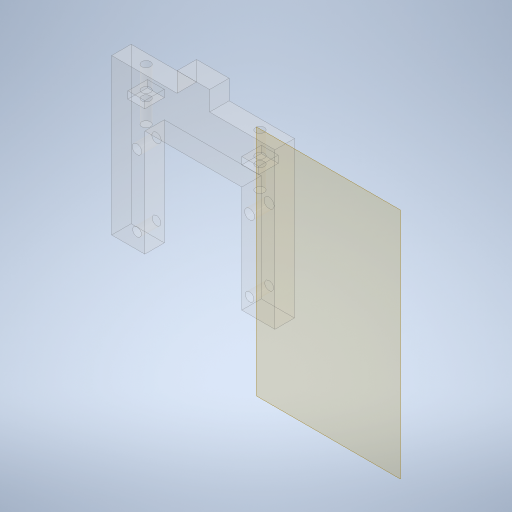
# Autodesk Inventor part: frame_knee_to_bridge
Saved by Autodesk Inventor 2024 (Build 280153000, 153)
## iProperties
Created: 2024-09-03
Part Number: frame_knee_to_bridge
Material: PMMA 플라스틱
Document SubType Name: Modeling
Designer: jmha0
Density: 1.188 g/cm^3
Appearance: 폴리카보네이트 - 선명
Mass: 4.02545 g
Surface Area: 28.6989 cm^2
Volume: 3.38842 cm^3
Author: jmha0
Autodesk Inventor part; units mm, degrees
ref_plane "YZ Plane" through (0, 0, 0) normal (1, 0, 0) x (0, 1, 0)
ref_plane "XZ Plane" through (0, 0, 0) normal (0, 1, 0) x (-1, 0, 0)
ref_plane "XY Plane" through (0, 0, 0) normal (0, 0, 1) x (1, 0, 0)
ref_plane "작업 평면1" through (0, 0, 0) normal (0, 0, 1) x (1, 0, 0)
sketch "스케치1" plane through (0, 0, 0) normal (0, 0, 1) x (1, 0, 0)
  line L0 (-20.1, 0.025) -> (-14.5, 0.025) projected
  line L1 (-20.1, -44.6) -> (-20.1, 8.5) projected
  line L2 (20.1, 0.025) -> (14.5, 0.025) projected
  line L3 (20.1, 8.5) -> (20.1, -44.6) projected
  circle A0 centre (17.3, 4) radius 1.45 projected
  circle A1 centre (-17.3, 4) radius 1.35 projected
  circle A2 centre (-17.3, 4) radius 1.45
  circle A3 centre (17.3, 4) radius 1.55
  line L4 (14.9, 0.025) -> (14.9, 15.025)
  line L5 (-14.9, 15.025) -> (-14.9, 0.025)
  line L6 (-20.1, 0.025) -> (-20.1, 15.025)
  line L7 (20.1, 0.025) -> (20.1, 15.025)
  line L8 (-20.1, 15.025) -> (20.1, 15.025)
  line L9 (-20.1, 0.025) -> (-14.9, 0.025)
  line L10 (14.9, 0.025) -> (20.1, 0.025)
  line L11 (-14.9, 0.025) -> (-14.9, 10.025)
  line L12 (-14.9, 10.025) -> (14.9, 10.025)
  line L13 (14.9, 0.025) -> (20.1, 0.025)
  point P0 (0, 0)
  point P1 (-20.1, 8.5)
  point P2 (-14.9, 0.025)
  dimension "d0" = 0.1
  dimension "d1" = 0.1
  dimension "d4" = 15
  dimension "d5" = 15
  dimension "d9" = 10
  constraints: 20 end point, 5 point on line, 2 centre point, 2 collinear, 2 perpendicular, 1 vertical
  measures "d0" radial gap between concentric circles of A1 A2
  measures "d1" radial gap between concentric circles of A0 A3
  measures "d4" distance of L0.start L6.end
  measures "d5" distance of L2.start L7.end
  measures "d9" distance of L5.end L11.end
extrude "돌출1" add sketch "스케치1" along normal blind 6 contours L1 L6 L8 L5 L0 | L5 L8 L4 L12 | L4 L8 L7 L3 L2
sketch "스케치5" plane through (0, 0, 6) normal (0, 0, 1) x (1, 0, 0)
  line L0 (15, -50.5) -> (11.5, -50.5)
  line L1 (15, -50.5) -> (20.1, -44.5)
  line L2 (20.1, -44.5) -> (20.1, 8.6)
  line L3 (20.1, 8.6) -> (15, 14.6)
  line L4 (15, 14.6) -> (-15, 14.6)
  line L5 (-15, 14.6) -> (-20.1, 8.6)
  line L6 (-20.1, 8.6) -> (-20.1, -44.5)
  line L7 (-20.1, -44.5) -> (-15, -50.5)
  line L8 (-11.5, -50.5) -> (-15, -50.5)
  arc A0 (-14.5, -47.5) -> (-11.5, -50.5) centre (-11.5, -47.5) ccw
  line L9 (-14.5, 6) -> (-14.5, -47.5)
  arc A1 (-11.5, 9) -> (-14.5, 6) centre (-11.5, 6) ccw
  line L10 (11.5, 9) -> (-11.5, 9)
  arc A2 (14.5, 6) -> (11.5, 9) centre (11.5, 6) ccw
  line L11 (14.5, -47.5) -> (14.5, 6)
  arc A3 (11.5, -50.5) -> (14.5, -47.5) centre (11.5, -47.5) ccw
  circle A4 centre (-17.3, -40) radius 1.35
  circle A5 centre (-17.3, -18) radius 1.35
  circle A6 centre (-17.3, 4) radius 1.35
  circle A7 centre (-11, 11.8) radius 1.35
  circle A8 centre (17.3, -40) radius 1.35
  circle A9 centre (17.3, -18) radius 1.35
  circle A10 centre (17.3, 4) radius 1.35
  circle A11 centre (11, 11.8) radius 1.35
  line L12 (20.1, 15.025) -> (-20.1, 15.025) projected
  line L13 (-20.1, 15.025) -> (-20.1, 0.025) projected
  line L14 (-20.1, 0.025) -> (-14.9, 0.025) projected
  line L15 (-14.9, 0.025) -> (-14.9, 10.025) projected
  line L16 (-14.9, 10.025) -> (14.9, 10.025) projected
  line L17 (14.9, 10.025) -> (14.9, 0.025) projected
  line L18 (14.9, 0.025) -> (20.1, 0.025) projected
  line L19 (20.1, 0.025) -> (20.1, 15.025) projected
  circle A12 centre (17.3, 4) radius 1.55 projected
  circle A13 centre (-17.3, 4) radius 1.45 projected
  line L20 (-14.9, 15.025) -> (-26.9, 15.025)
  line L21 (-26.9, 15.025) -> (-26.9, -22.7435)
  line L22 (-26.9, -22.7435) -> (-14.9, -22.7435)
  line L23 (-14.9, -22.7435) -> (-14.9, 15.025)
  line L24 (14.9, 15.025) -> (26.9, 15.025)
  line L25 (26.9, 15.025) -> (26.9, -22.7435)
  line L26 (26.9, -22.7435) -> (14.9, -22.7435)
  line L27 (14.9, -22.7435) -> (14.9, 15.025)
  point P0 (0, 0)
  point P1 (0, -36)
  point P2 (20.1, 8.6)
  point P3 (20.1, -22.7435)
  point P4 (-20.1, -22.7435)
  point P5 (-20.1, 15.025)
  point P6 (20.1, 0.025)
  point P7 (-14.9, 0.025)
  dimension "d21" = 12
  dimension "d22" = 12
  constraints: 40 end point, 12 centre point, 8 point on circle, 4 parallel, 2 perpendicular, 2 point on line
  measures "d21" distance of L20.start L20.end
  measures "d22" distance of L24.start L24.end
extrude "돌출5" add sketch "스케치5" against normal blind 6 contours L26 L27 L18 L2 | L23 L22 L6 L14
sketch "스케치12" plane through (0, 0, 6) normal (0, 0, 1) x (1, 0, 0)
  circle A0 centre (-17.3, -18) radius 1.35 projected
  circle A1 centre (17.3, -18) radius 1.35 projected
  line L0 (20.1, 15.025) -> (-20.1, 15.025) projected
  line L1 (-20.1, 15.025) -> (-20.1, -22.7435) projected
  line L2 (-20.1, -22.7435) -> (-14.9, -22.7435) projected
  line L3 (-14.9, -22.7435) -> (-14.9, 10.025) projected
  line L4 (-14.9, 10.025) -> (14.9, 10.025) projected
  line L5 (14.9, 10.025) -> (14.9, -22.7435) projected
  line L6 (14.9, -22.7435) -> (20.1, -22.7435) projected
  line L7 (20.1, -22.7435) -> (20.1, 15.025) projected
  circle A2 centre (17.3, 4) radius 1.55 projected
  circle A3 centre (-17.3, 4) radius 1.45 projected
  line L8 (0, 15.025) -> (-5, 15.025)
  line L9 (-5, 15.025) -> (-5, 21.025)
  line L10 (-5, 21.025) -> (0, 21.025)
  line L11 (0, 21.025) -> (0, 15.025)
  line L12 (0, 21.025) -> (5, 21.025)
  line L13 (5, 21.025) -> (5, 15.025)
  line L14 (5, 15.025) -> (0, 15.025)
  line L15 (0, 15.025) -> (0, 21.025)
  point P0 (0, 0)
  point P1 (5, 15.025)
  dimension "d53" = 5
  dimension "d54" = 6
  dimension "d55" = 5
  dimension "d56" = 6
  constraints: 16 end point, 4 parallel, 2 horizontal, 2 perpendicular, 1 midpoint
  measures "d53" distance of L9.end L10.end
  measures "d54" distance of L8.end L9.end
  measures "d55" distance of L13.end L14.end
  measures "d56" distance of L12.end L13.end
extrude "돌출11" add sketch "스케치12" against normal blind 6 contours L0 L11 L12 L13 | L0 L9 L10 L11
sketch "스케치14" plane through (-20.1, 15.025, 6) normal (0, 1, 0) x (1, 0, 0)
  line L0 (5.2, 6) -> (5.2, 0) projected
  line L1 (15.1, 0) -> (15.1, 6) projected
  line L2 (15.1, 6) -> (0, 6) projected
  line L3 (0, 6) -> (0, 0) projected
  line L4 (15.1, 0) -> (0, 0) projected
  line L5 (25.1, 6) -> (25.1, 0) projected
  line L6 (40.2, 0) -> (25.1, 0) projected
  line L7 (40.2, 6) -> (40.2, 0) projected
  line L8 (40.2, 6) -> (25.1, 6) projected
  line L9 (35, 6) -> (35, 0) projected
  line L10 (0, 6) -> (2.6, 6)
  circle A0 centre (2.6, 3) radius 1.35
  line L11 (40.2, 6) -> (40.2, 0) projected
  line L12 (40.2, 6) -> (37.6, 6)
  circle A1 centre (37.6, 3) radius 1.35
  point P0 (20.1, 6)
  dimension "d59" = 6
  dimension "d60" = 5.2
  dimension "d61" = 2.6
  dimension "d62" = 2.7
  dimension "d63" = 2.6
  dimension "d64" = 2.7
  constraints: 4 end point, 2 centre point, 2 point on line
  measures "d59" distance of L2.end L3.end
  measures "d60" distance between parallel lines of L0 L3
  measures "d61" distance of L2.end L10.end
  measures "d62" diameter of A0
  measures "d63" distance of L7.start L12.end
  measures "d64" diameter of A1
extrude "돌출12" cut sketch "스케치14" against normal blind 6 contours A0 | A1
sketch "스케치16" plane through (-20.1, 15.025, 0) normal (-1, 0, 0) x (0, 0, 1)
  line L0 (0, 0) -> (0, -37.7685) projected
  line L1 (6, -37.7685) -> (0, -37.7685) projected
  line L2 (6, 0) -> (6, -37.7685) projected
  line L3 (0, 0) -> (6, 0) projected
  point P0 (0, -15.025)
extrude "돌출13" add sketch "스케치16" along normal blind 5
sketch "스케치18" plane through (20.1, 15.025, 6) normal (1, 0, 0) x (0, 0, -1)
  line L0 (6, 0) -> (6, -37.7685) projected
  line L1 (6, 0) -> (0, 0) projected
  line L2 (0, -37.7685) -> (0, 0) projected
  line L3 (0, -37.7685) -> (6, -37.7685) projected
  point P0 (6, -15.025)
extrude "돌출14" add sketch "스케치18" along normal blind 5
move faces "이동1" translate (0, 10, 0) faces at (8.7167, 15.025, 3) (1.6667, 21.025, 4) (-8.7167, 15.025, 3)
sketch "스케치19" plane through (0, 0, 6) normal (0, 0, 1) x (1, 0, 0)
  line L0 (-18.85, 9.025) -> (-16.15, 9.025) projected
  circle A0 centre (-17.3, 4) radius 1.45 projected
  line L1 (-14.9, 10.025) -> (14.9, 10.025) projected
  line L2 (-14.9, 10.025) -> (14.9, 10.025) projected
  circle A1 centre (-17.3, -18) radius 1.35 projected
  circle A2 centre (17.3, -18) radius 1.35 projected
  line L3 (5, 25.025) -> (25.1, 25.025) projected
  line L4 (5, 25.025) -> (5, 31.025) projected
  line L5 (5, 31.025) -> (-5, 31.025) projected
  line L6 (-5, 31.025) -> (-5, 25.025) projected
  line L7 (-5, 25.025) -> (-25.1, 25.025) projected
  line L8 (-25.1, -22.7435) -> (-25.1, 25.025) projected
  line L9 (-25.1, -22.7435) -> (-14.9, -22.7435) projected
  line L10 (-14.9, -22.7435) -> (-14.9, 10.025) projected
  line L11 (-14.9, 10.025) -> (14.9, 10.025) projected
  line L12 (14.9, 10.025) -> (14.9, -22.7435) projected
  line L13 (14.9, -22.7435) -> (25.1, -22.7435) projected
  line L14 (25.1, 25.025) -> (25.1, -22.7435) projected
  circle A3 centre (17.3, 4) radius 1.55 projected
  circle A4 centre (-17.3, 4) radius 1.45 projected
  circle A5 centre (-17.3, -18) radius 1.35 projected
  circle A6 centre (17.3, -18) radius 1.35 projected
  line L15 (25.1, 25.025) -> (5, 25.025) projected
  line L16 (25.1, -22.7435) -> (25.1, 25.025) projected
  line L17 (14.9, -22.7435) -> (25.1, -22.7435) projected
  line L18 (14.9, 10.025) -> (14.9, -22.7435) projected
  line L19 (-14.9, 10.025) -> (14.9, 10.025) projected
  line L20 (-14.9, 10.025) -> (-14.9, -22.7435) projected
  line L21 (-14.9, -22.7435) -> (-25.1, -22.7435) projected
  line L22 (-25.1, 25.025) -> (-25.1, -22.7435) projected
  line L23 (-5, 25.025) -> (-25.1, 25.025) projected
  line L24 (-5, 25.025) -> (-5, 31.025) projected
  line L25 (-5, 31.025) -> (5, 31.025) projected
  line L26 (5, 31.025) -> (5, 25.025) projected
  circle A7 centre (17.3, 4) radius 1.55 projected
  circle A8 centre (-17.3, 4) radius 1.45 projected
  line L27 (-5, 25.025) -> (-5, 31.025) projected
  line L28 (-14.9, -22.7435) -> (-14.9, 10.025) projected
  line L29 (-14.9, 10.025) -> (-14.9, -22.7435) projected
  line L30 (-14.9, 10.025) -> (-14.9, -22.7435) projected
  line L31 (-14.9, -22.7435) -> (-14.9, 10.025) projected
  circle A9 centre (-17.3, -18) radius 1.35 projected
  circle A10 centre (-17.3, -18) radius 1.35 projected
  circle A11 centre (-17.3, -18) radius 1.35 projected
  circle A12 centre (-17.3, -18) radius 1.35 projected
  circle A13 centre (-17.3, 4) radius 1.45 projected
  circle A14 centre (-17.3, 4) radius 1.45 projected
  circle A15 centre (-17.3, 4) radius 1.45 projected
  line L32 (-25.1, -22.7435) -> (-14.9, -22.7435) projected
  line L33 (-14.9, -22.7435) -> (-25.1, -22.7435) projected
  line L34 (-25.1, -22.7435) -> (-14.9, -22.7435) projected
  line L35 (-14.9, -22.7435) -> (-25.1, -22.7435) projected
  line L36 (-25.1, -22.7435) -> (-25.1, 25.025) projected
  line L37 (-25.1, 25.025) -> (-25.1, -22.7435) projected
  line L38 (-25.1, 25.025) -> (-25.1, -22.7435) projected
  line L39 (-25.1, -22.7435) -> (-25.1, 25.025) projected
  line L40 (14.9, -22.7435) -> (25.1, -22.7435) projected
  line L41 (14.9, 10.025) -> (14.9, -22.7435) projected
  line L42 (14.9, 10.025) -> (14.9, -22.7435) projected
  circle A16 centre (17.3, -18) radius 1.35 projected
  circle A17 centre (17.3, -18) radius 1.35 projected
  circle A18 centre (17.3, 4) radius 1.55 projected
  circle A19 centre (17.3, 4) radius 1.55 projected
  line L43 (16.15, 9.025) -> (18.85, 9.025) projected
  line L44 (14.9, -22.7435) -> (25.1, -22.7435) projected
  line L45 (25.1, 25.025) -> (25.1, -22.7435) projected
  line L46 (25.1, -22.7435) -> (25.1, 25.025) projected
  line L47 (25.1, -22.7435) -> (25.1, 25.025) projected
  line L48 (25.1, 25.025) -> (25.1, -22.7435) projected
  line L49 (-18.85, 9.025) -> (-16.15, 9.025) projected
  line L50 (-18.85, 25.025) -> (-16.15, 25.025) projected
  line L51 (-18.85, 9.025) -> (-16.15, 9.025) projected
  line L52 (-5, 25.025) -> (-25.1, 25.025) projected
  line L53 (-5, 25.025) -> (-25.1, 25.025) projected
  line L54 (-18.85, 25.025) -> (-16.15, 25.025) projected
  line L55 (-5, 25.025) -> (-25.1, 25.025) projected
  line L56 (-5, 25.025) -> (-25.1, 25.025) projected
  line L57 (-5, 31.025) -> (-5, 25.025) projected
  line L58 (5, 31.025) -> (-5, 31.025) projected
  line L59 (5, 31.025) -> (-5, 31.025) projected
  line L60 (-5, 31.025) -> (5, 31.025) projected
  line L61 (-5, 31.025) -> (-5, 25.025) projected
  line L62 (-5, 25.025) -> (-5, 31.025) projected
  line L63 (-18.85, 25.025) -> (-16.15, 25.025) projected
  line L64 (16.15, 25.025) -> (18.85, 25.025) projected
  line L65 (5, 25.025) -> (25.1, 25.025) projected
  line L66 (25.1, 25.025) -> (5, 25.025) projected
  line L67 (5, 31.025) -> (5, 25.025) projected
  line L68 (5, 25.025) -> (5, 31.025) projected
  line L69 (5, 25.025) -> (5, 31.025) projected
  line L70 (5, 31.025) -> (5, 25.025) projected
  line L71 (-5, 31.025) -> (5, 31.025) projected
  line L72 (14.9, -22.7435) -> (25.1, -22.7435) projected
  line L73 (14.9, -22.7435) -> (25.1, -22.7435) projected
  line L74 (-14.9, 10.025) -> (14.9, 10.025) projected
  line L75 (-14.9, 10.025) -> (14.9, 10.025) projected
  circle A20 centre (17.3, -18) radius 1.35 projected
  circle A21 centre (17.3, -18) radius 1.35 projected
  line L76 (14.9, 10.025) -> (14.9, -22.7435) projected
  line L77 (14.9, 10.025) -> (14.9, -22.7435) projected
  line L78 (16.15, 9.025) -> (18.85, 9.025) projected
  line L79 (16.15, 25.025) -> (18.85, 25.025) projected
  line L80 (16.15, 25.025) -> (18.85, 25.025) projected
  line L81 (5, 25.025) -> (25.1, 25.025) projected
  line L82 (25.1, 25.025) -> (5, 25.025) projected
  circle A22 centre (17.3, 4) radius 1.55 projected
  circle A23 centre (17.3, 4) radius 1.55 projected
  line L83 (16.15, 9.025) -> (18.85, 9.025) projected
  line L84 (-18.85, 25.025) -> (-18.85, 9.025) projected
  line L85 (-16.15, 25.025) -> (-16.15, 9.025) projected
  line L86 (16.15, 25.025) -> (16.15, 9.025) projected
  line L87 (18.85, 25.025) -> (18.85, 9.025) projected
  line L88 (-20.1, 15.925) -> (-14.9, 15.925)
  line L89 (-14.9, 15.925) -> (-14.9, 18.125)
  line L90 (-14.9, 18.125) -> (-20.1, 18.125)
  line L91 (-20.1, 18.125) -> (-20.1, 15.925)
  line L92 (-20.1, 15.925) -> (-14.9, 18.125) construction
  line L93 (-14.9, 15.925) -> (-20.1, 18.125) construction
  line L94 (14.9, 15.925) -> (20.1, 15.925)
  line L95 (20.1, 15.925) -> (20.1, 18.125)
  line L96 (20.1, 18.125) -> (14.9, 18.125)
  line L97 (14.9, 18.125) -> (14.9, 15.925)
  line L98 (14.9, 15.925) -> (20.1, 18.125) construction
  line L99 (20.1, 15.925) -> (14.9, 18.125) construction
  point P0 (0, 0)
  point P1 (-17.5, 17.025)
  point P2 (17.5, 17.025)
  dimension "d74" = 5.2
  dimension "d75" = 2.2
  dimension "d76" = 5.2
  dimension "d77" = 2.2
  constraints: 24 end point, 4 midpoint, 4 parallel, 2 horizontal, 2 perpendicular, 1 other
  measures "d74" distance of L90.end L89.end
  measures "d75" distance of L89.end L88.end
  measures "d76" distance of L96.end L95.end
  measures "d77" distance of L95.end L94.end
extrude "돌출15" cut sketch "스케치19" against normal blind 10 contours L88 L91 L90 L84 | L84 L90 L85 L88 | L85 L90 L89 L88 | L96 L87 L94 L86 | L86 L94 L97 L96 | L96 L95 L94 L87
